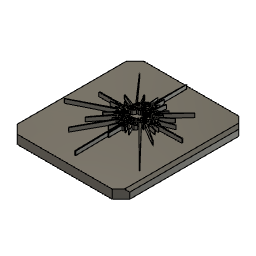
Plaque Nomai (Autodesk Fusion 360 design; units mm, degrees)
Autodesk Fusion 360 part; units mm, degrees
sketch "Sketch1" plane through (0, 0, 0) normal (0, 1, 0) x (1, 0, 0)
  line L0 (0, 0) -> (16, 0)
  line L1 (16, 0) -> (16, -18)
  line L2 (16, -18) -> (0, -18)
  line L3 (0, -18) -> (0, 0)
  constraint horizontal L0
  constraint vertical L1
  constraint horizontal L2
  constraint vertical L3
  constraint coincident L0.start L3.end
extrude "Extrude1" add sketch "Sketch1" along normal blind 3 contours L0 L1 L2 L3 picked at (5.333333, -12) makes body 1
sketch "Sketch2" plane through (0, 3, 0) normal (0, 1, 0) x (-1, 0, 0)
  line L0 (-3.5, 4) -> (-3.55, 4)
  line L1 (-3.55, 4) -> (-6.6, 7.39)
  line L2 (-6.6, 7.39) -> (-6.783242, 7.248473)
  line L3 (-6.783242, 7.248473) -> (-7.45, 7.248473)
  line L4 (-7.45, 7.248473) -> (-7.5, 7.45)
  line L5 (-7.5, 7.45) -> (-7.55, 7.45)
  line L6 (-7.55, 7.45) -> (-7.55, 7.15)
  line L7 (-7.55, 7.15) -> (-7.66975, 7.15)
  line L8 (-7.66975, 7.15) -> (-7.7, 7.6)
  line L9 (-7.7, 7.6) -> (-7.348129, 7.623653)
  line L10 (-7.348129, 7.623653) -> (-7.331455, 7.3756)
  line L11 (-7.331455, 7.3756) -> (-6.800321, 7.388831)
  line L12 (-6.800321, 7.388831) -> (-6.608305, 7.559685)
  line L13 (-6.608305, 7.559685) -> (-3.5, 4)
  line L14 (-6.2, 6.1) -> (-6.258087, 6.047739)
  line L15 (-6.258087, 6.047739) -> (-6.9, 7)
  line L16 (-6.9, 7) -> (-6.95, 7)
  line L17 (-6.95, 7) -> (-7.345894, 6.643813)
  line L18 (-7.345894, 6.643813) -> (-7.382435, 6.821906)
  line L19 (-7.382435, 6.821906) -> (-7.025574, 7.142976)
  line L20 (-7.025574, 7.142976) -> (-6.85, 7.142976)
  line L21 (-6.85, 7.142976) -> (-6.2, 6.1)
  line L22 (-7.191091, 7.142976) -> (-7.4, 7.142976)
  line L23 (-7.4, 7.142976) -> (-7.593291, 6.848491)
  line L24 (-7.593291, 6.848491) -> (-7.4, 5.527504)
  line L25 (-7.4, 5.527504) -> (-7.496646, 6.821906)
  line L26 (-7.496646, 6.821906) -> (-7.191091, 7.142976)
  line L27 (-7.609875, 7.047702) -> (-7.879433, 7.047702)
  line L28 (-7.879433, 7.047702) -> (-7.83, 2.2)
  line L29 (-7.83, 2.2) -> (-7.794916, 2.200358)
  line L30 (-7.794916, 2.200358) -> (-7.716057, 6.848491)
  line L31 (-7.716057, 6.848491) -> (-7.609875, 7.047702)
  line L32 (-8, 6.6) -> (-8.3, 6.6)
  line L33 (-8.3, 6.6) -> (-8.339414, 6.187997)
  line L34 (-8.339414, 6.187997) -> (-8.244092, 6.499241)
  line L35 (-8.244092, 6.499241) -> (-8.06588, 6.499241)
  line L36 (-8.06588, 6.499241) -> (-8.06588, 5.342936)
  line L37 (-8.06588, 5.342936) -> (-8, 5.342936)
  line L38 (-8, 5.342936) -> (-8, 6.6)
  line L39 (-8.438881, 7.087755) -> (-8.708271, 5.753238)
  line L40 (-8.708271, 5.753238) -> (-8.764863, 5.764661)
  line L41 (-8.764863, 5.764661) -> (-8.573576, 7.141633)
  line L42 (-8.573576, 7.141633) -> (-8.438881, 7.087755)
  line L43 (-8, 6.7) -> (-8.35, 6.7)
  line L44 (-8.35, 6.7) -> (-8.35, 7.2)
  line L45 (-8.35, 7.2) -> (-8.6, 7.2)
  line L46 (-8.6, 7.2) -> (-8.8, 6.95)
  line L47 (-8.8, 6.95) -> (-8.980246, 7.056907)
  line L48 (-8.980246, 7.056907) -> (-9.60392, 6.277315)
  line L49 (-9.60392, 6.277315) -> (-9.637964, 6.30455)
  line L50 (-9.637964, 6.30455) -> (-9.013716, 7.247048)
  line L51 (-9.013716, 7.247048) -> (-8.890123, 7.165188)
  line L52 (-8.890123, 7.165188) -> (-8.74056, 7.352142)
  line L53 (-8.74056, 7.352142) -> (-8.248844, 7.352142)
  line L54 (-8.248844, 7.352142) -> (-8.248844, 6.868399)
  line L55 (-8.248844, 6.868399) -> (-8, 6.868399)
  line L56 (-8, 6.868399) -> (-8, 6.7)
  line L57 (-8.001395, 6.96448) -> (-8.142811, 6.96448)
  line L58 (-8.142811, 6.96448) -> (-8.142811, 7.354078)
  line L59 (-8.142811, 7.354078) -> (-7.92088, 7.354078)
  line L60 (-7.92088, 7.354078) -> (-7.92088, 7.975797)
  line L61 (-7.92088, 7.975797) -> (-7.801013, 7.975797)
  line L62 (-7.801013, 7.975797) -> (-7.758384, 7.156414)
  line L63 (-7.758384, 7.156414) -> (-8, 7.156414)
  line L64 (-8, 7.156414) -> (-8.001395, 6.96448)
  line L65 (-8, 8.1) -> (-8.004849, 7.433169)
  line L66 (-8.004849, 7.433169) -> (-9.03, 7.41)
  line L67 (-9.03, 7.41) -> (-11.530001, 4.85)
  line L68 (-11.530001, 4.85) -> (-11.550001, 4.89)
  line L69 (-11.550001, 4.89) -> (-9.09, 7.54)
  line L70 (-9.09, 7.54) -> (-8.14, 7.56)
  line L71 (-8.14, 7.56) -> (-8.14, 8.15)
  line L72 (-8.14, 8.15) -> (-8, 8.1)
  line L73 (-8.25, 7.65) -> (-8.25, 8)
  line L74 (-8.25, 8) -> (-8.65, 7.65)
  line L75 (-8.65, 7.65) -> (-8.25, 7.65)
  line L76 (-8.25, 8.15) -> (-8.8, 7.65)
  line L77 (-8.8, 7.65) -> (-9.3, 8.15)
  line L78 (-9.3, 8.15) -> (-9.22, 8.25)
  line L79 (-9.22, 8.25) -> (-8.795, 7.825)
  line L80 (-8.795, 7.825) -> (-8.4375, 8.15)
  line L81 (-8.4375, 8.15) -> (-8.25, 8.15)
  line L82 (-8.4, 8.35) -> (-8.795, 7.955)
  line L83 (-8.795, 7.955) -> (-8.901457, 8.061457)
  line L84 (-8.901457, 8.061457) -> (-8.488611, 8.474303)
  line L85 (-8.488611, 8.474303) -> (-8.4, 8.35)
  line L86 (-8.546308, 8.555239) -> (-8.949047, 8.1525)
  line L87 (-8.949047, 8.1525) -> (-9.02, 8.21)
  line L88 (-9.02, 8.21) -> (-8.7, 8.55)
  line L89 (-8.7, 8.55) -> (-8.546308, 8.555239)
  line L90 (-9.075018, 7.787234) -> (-9.352052, 8.091971)
  line L91 (-9.352052, 8.091971) -> (-9.459599, 7.994201)
  line L92 (-9.459599, 7.994201) -> (-9.267314, 7.774446)
  line L93 (-9.267314, 7.774446) -> (-9.773316, 7.164174)
  line L94 (-9.773316, 7.164174) -> (-9.711912, 7.113262)
  line L95 (-9.711912, 7.113262) -> (-9.075018, 7.787234)
  line L96 (-8.945038, 7.644256) -> (-9.018767, 7.713929)
  line L97 (-9.018767, 7.713929) -> (-9.075018, 7.644256)
  line L98 (-9.075018, 7.644256) -> (-8.945038, 7.644256)
  line L99 (-8.8294, 8.584728) -> (-9.3, 8.584728)
  line L100 (-9.3, 8.584728) -> (-9.794941, 7.973993)
  line L101 (-9.794941, 7.973993) -> (-9.75, 7.75)
  line L102 (-9.75, 7.75) -> (-10.910001, 6.75)
  line L103 (-10.910001, 6.75) -> (-10.883433, 6.719182)
  line L104 (-10.883433, 6.719182) -> (-10.874451, 6.720984)
  line L105 (-9.54, 7.73) -> (-10.874451, 6.720984)
  line L106 (-9.54, 7.73) -> (-9.594657, 7.939603)
  line L107 (-9.594657, 7.939603) -> (-9.213535, 8.371845)
  line L108 (-9.213535, 8.371845) -> (-9.1, 8.28)
  line L109 (-9.1, 8.28) -> (-8.8294, 8.584728)
  line L110 (-9.757394, 8.193299) -> (-9.898058, 8.019727)
  line L111 (-9.898058, 8.019727) -> (-11.680001, 7.43)
  line L112 (-11.680001, 7.43) -> (-11.691706, 7.465371)
  line L113 (-11.691706, 7.465371) -> (-10.02, 8.13)
  line L114 (-10.02, 8.13) -> (-10.060088, 8.251131)
  line L115 (-10.060088, 8.251131) -> (-10.069408, 8.279292)
  line L116 (-10.069408, 8.279292) -> (-10.523963, 8.301132)
  line L117 (-10.523963, 8.301132) -> (-10.522401, 8.333643)
  line L118 (-10.522401, 8.333643) -> (-9.998681, 8.411924)
  line L119 (-9.998681, 8.411924) -> (-9.757394, 8.193299)
  line L120 (-9.696027, 8.279361) -> (-9.952526, 8.529848)
  line L121 (-9.952526, 8.529848) -> (-13.6, 8.5)
  line L122 (-13.6, 8.5) -> (-13.600686, 8.583817)
  line L123 (-13.600686, 8.583817) -> (-9.880537, 8.680784)
  line L124 (-9.880537, 8.680784) -> (-9.62, 8.38)
  line L125 (-9.62, 8.38) -> (-9.696027, 8.279361)
  line L126 (-9.479969, 8.54549) -> (-9.556698, 8.465692)
  line L127 (-9.556698, 8.465692) -> (-9.856172, 8.784172)
  line L128 (-9.856172, 8.784172) -> (-10.840001, 8.84)
  line L129 (-10.840001, 8.84) -> (-10.860001, 8.89)
  line L130 (-10.860001, 8.89) -> (-9.814413, 8.89)
  line L131 (-9.814413, 8.89) -> (-9.479969, 8.54549)
  line L132 (-9.518334, 8.758434) -> (-9.518334, 9.170027)
  line L133 (-9.518334, 9.170027) -> (-9.929882, 9.170027)
  line L134 (-9.929882, 9.170027) -> (-10.9, 9.4)
  line L135 (-10.9, 9.4) -> (-10.911903, 9.349787)
  line L136 (-10.911903, 9.349787) -> (-10, 9)
  line L137 (-10, 9) -> (-9.7, 9)
  line L138 (-9.7, 9) -> (-9.7, 8.939707)
  line L139 (-9.7, 8.939707) -> (-9.518334, 8.758434)
  line L140 (-8.537747, 8.691775) -> (-9.439601, 8.691775)
  line L141 (-9.439601, 8.691775) -> (-9.439601, 9.156301)
  line L142 (-9.439601, 9.156301) -> (-8.413887, 9.170027)
  line L143 (-8.537747, 8.691775) -> (-8.537747, 8.761446)
  line L144 (-8.537747, 8.761446) -> (-9.3, 8.8)
  line L145 (-9.3, 8.8) -> (-9.314788, 8.99633)
  line L146 (-9.314788, 8.99633) -> (-8.483616, 9.023874)
  line L147 (-8.483616, 9.023874) -> (-8.413887, 9.170027)
  line L148 (-8.523626, 8.940011) -> (-9.214555, 8.917115)
  line L149 (-9.214555, 8.917115) -> (-9.213155, 8.874853)
  line L150 (-9.213155, 8.874853) -> (-8.564151, 8.85507)
  line L151 (-8.564151, 8.85507) -> (-8.523626, 8.940011)
  line L152 (-8.459454, 9.588483) -> (-8.838801, 9.23942)
  line L153 (-8.838801, 9.23942) -> (-9.769123, 9.23942)
  line L154 (-9.769123, 9.23942) -> (-12.025575, 10.717433)
  line L155 (-12.025575, 10.717433) -> (-11.99598, 10.762616)
  line L156 (-11.99598, 10.762616) -> (-9.638536, 9.38846)
  line L157 (-9.638536, 9.38846) -> (-8.95, 9.38846)
  line L158 (-8.95, 9.38846) -> (-8.460762, 9.890243)
  line L159 (-8.460762, 9.890243) -> (-8.459454, 9.588483)
  line L160 (-8.95, 9.5) -> (-9.25, 9.5)
  line L161 (-9.25, 9.5) -> (-14.004695, 14.440687)
  line L162 (-14.004695, 14.440687) -> (-13.960001, 14.470001)
  line L163 (-13.960001, 14.470001) -> (-8.95, 9.5)
  line L164 (-9.415286, 9.5) -> (-9.554376, 9.5)
  line L165 (-9.554376, 9.5) -> (-9.590117, 9.537139)
  line L166 (-9.590117, 9.537139) -> (-9.554376, 9.595452)
  line L167 (-9.554376, 9.595452) -> (-9.415286, 9.5)
  line L168 (-8.5, 10) -> (-8.861207, 9.595452)
  line L169 (-8.861207, 9.595452) -> (-9.087752, 9.797726)
  line L170 (-9.087752, 9.797726) -> (-8.974479, 9.924589)
  line L171 (-8.974479, 9.924589) -> (-8.893129, 9.797726)
  line L172 (-8.893129, 9.797726) -> (-8.723811, 9.98736)
  line L173 (-8.723811, 9.98736) -> (-8.5, 10)
  line L174 (-8.515772, 9.833823) -> (-8.460762, 9.890243)
  line L175 (-8.350321, 9.702011) -> (-8.238397, 9.702496)
  line L176 (-8.238397, 9.702496) -> (-8.240191, 10.116471)
  line L177 (-8.240191, 10.116471) -> (-8.4, 10.2)
  line L178 (-8.4, 10.2) -> (-9.017739, 10.197322)
  line L179 (-9.017739, 10.197322) -> (-9.252195, 9.960979)
  line L180 (-9.252195, 9.960979) -> (-9.177243, 9.886625)
  line L181 (-9.177243, 9.886625) -> (-8.961542, 10.104062)
  line L182 (-8.961542, 10.104062) -> (-8.396178, 10.106512)
  line L183 (-8.396178, 10.106512) -> (-8.368597, 10.079151)
  line L184 (-8.368597, 10.079151) -> (-8.350321, 9.702011)
  line L185 (-8.320095, 10.48169) -> (-8.46955, 10.314302)
  line L186 (-8.46955, 10.314302) -> (-8.874608, 10.314302)
  line L187 (-8.874608, 10.314302) -> (-9.267118, 11.085337)
  line L188 (-9.267118, 11.085337) -> (-9.227774, 11.129402)
  line L189 (-9.227774, 11.129402) -> (-8.70887, 10.494309)
  line L190 (-8.70887, 10.494309) -> (-8.320095, 10.48169)
  line L191 (-8.218928, 10.594995) -> (-8.572943, 10.593461)
  line L192 (-8.572943, 10.593461) -> (-8.778364, 11.076791)
  line L193 (-8.778364, 11.076791) -> (-8.778648, 11.142484)
  line L194 (-8.778648, 11.142484) -> (-8.514482, 10.738211)
  line L195 (-8.514482, 10.738211) -> (-8.25, 10.7)
  line L196 (-8.25, 10.7) -> (-8.2, 10.75)
  line L197 (-8.2, 10.75) -> (-8.225, 12.675482)
  line L198 (-8.225, 12.675482) -> (-8.173235, 12.727247)
  line L199 (-8.173235, 12.727247) -> (-8.142708, 12.675482)
  line L200 (-8.142708, 12.675482) -> (-8.1, 10.7)
  line L201 (-8.1, 10.7) -> (-8.218928, 10.594995)
  line L202 (-8.329908, 10.828133) -> (-8.416009, 10.840573)
  line L203 (-8.416009, 10.840573) -> (-8.461558, 10.932274)
  line L204 (-8.461558, 10.932274) -> (-8.309915, 11.066163)
  line L205 (-8.309915, 11.066163) -> (-8.30891, 10.834353)
  line L206 (-8.30891, 10.834353) -> (-8.329908, 10.828133)
  line L207 (-8.05, 9.5) -> (-8.35, 9.5)
  line L208 (-8.35, 9.5) -> (-8.351472, 9.609975)
  line L209 (-8.351472, 9.609975) -> (-8.2, 9.609975)
  line L210 (-8.2, 9.609975) -> (-8.16102, 9.638167)
  line L211 (-8.16102, 9.638167) -> (-8.16102, 10.128527)
  line L212 (-8.16102, 10.128527) -> (-8.05, 10.25)
  line L213 (-8.05, 10.25) -> (-8.05, 9.5)
  line L214 (-7.7, 9.75) -> (-7.85, 9.75)
  line L215 (-7.85, 9.75) -> (-7.85, 9.35)
  line L216 (-7.85, 9.35) -> (-8.05, 9.35)
  line L217 (-8.05, 9.35) -> (-8.25, 9.25)
  line L218 (-8.25, 9.25) -> (-8.65, 9.25)
  line L219 (-8.65, 9.25) -> (-8.5, 9.4)
  line L220 (-8.5, 9.4) -> (-8, 9.4)
  line L221 (-8, 9.4) -> (-7.95, 9.4)
  line L222 (-7.95, 9.4) -> (-7.975, 9.93339)
  line L223 (-7.975, 9.93339) -> (-7.687787, 9.946851)
  line L224 (-7.687787, 9.946851) -> (-7.7, 9.75)
  line L225 (-8.23, 10.22) -> (-8.310655, 10.293715)
  line L226 (-8.310655, 10.293715) -> (-8.002551, 10.630825)
  line L227 (-8.002551, 10.630825) -> (-8.10551, 16.826528)
  line L228 (-8.10551, 16.826528) -> (-8.002551, 16.843181)
  line L229 (-8.002551, 16.843181) -> (-7.898695, 10.593466)
  line L230 (-7.898695, 10.593466) -> (-8.23, 10.22)
  line L231 (-7.713999, 9.524356) -> (-7.524068, 9.512573)
  line L232 (-7.524068, 9.512573) -> (-7.45, 9.55)
  line L233 (-7.45, 9.55) -> (-7.487034, 10.167916)
  line L234 (-7.487034, 10.167916) -> (-7.8, 10.167916)
  line L235 (-7.8, 10.167916) -> (-7.805924, 10.266755)
  line L236 (-7.805924, 10.266755) -> (-7.598199, 10.505373)
  line L237 (-7.598199, 10.505373) -> (-7.622996, 10.919112)
  line L238 (-7.622996, 10.919112) -> (-7.308455, 11.817933)
  line L239 (-7.308455, 11.817933) -> (-7.359161, 11.862073)
  line L240 (-7.359161, 11.862073) -> (-7.783134, 10.919112)
  line L241 (-7.783134, 10.919112) -> (-7.777477, 10.57874)
  line L242 (-7.777477, 10.57874) -> (-7.950623, 10.365557)
  line L243 (-7.950623, 10.365557) -> (-7.950623, 10.029722)
  line L244 (-7.950623, 10.029722) -> (-7.619829, 10.029722)
  line L245 (-7.619829, 10.029722) -> (-7.596455, 9.700116)
  line L246 (-7.596455, 9.700116) -> (-7.643517, 9.646055)
  line L247 (-7.643517, 9.646055) -> (-7.748004, 9.673086)
  line L248 (-7.748004, 9.673086) -> (-7.713999, 9.524356)
  line L249 (-7.266689, 10.801328) -> (-7.425065, 10.518635)
  line L250 (-7.425065, 10.518635) -> (-7.515354, 10.517134)
  line L251 (-7.515354, 10.517134) -> (-7.521353, 10.878116)
  line L252 (-7.521353, 10.878116) -> (-7.458429, 10.990431)
  line L253 (-7.458429, 10.990431) -> (-7.266689, 10.801328)
  line L254 (-7.324009, 10.180051) -> (-7.415948, 10.174541)
  line L255 (-7.415948, 10.174541) -> (-7.408061, 10.042959)
  line L256 (-7.408061, 10.042959) -> (-7.324009, 10.180051)
  line L257 (-7.256565, 10.290054) -> (-7.658368, 10.265973)
  line L258 (-7.658368, 10.265973) -> (-7.559894, 10.426586)
  line L259 (-7.559894, 10.426586) -> (-7.369978, 10.426586)
  line L260 (-7.369978, 10.426586) -> (-5.028617, 14.663257)
  line L261 (-5.028617, 14.663257) -> (-4.952926, 14.621427)
  line L262 (-4.952926, 14.621427) -> (-7.256565, 10.290054)
  line L263 (-6.70707, 9.928836) -> (-7.07594, 10.360941)
  line L264 (-7.07594, 10.360941) -> (-6.736052, 10.75616)
  line L265 (-6.736052, 10.75616) -> (-6.692551, 10.732119)
  line L266 (-6.692551, 10.732119) -> (-6.891505, 10.372115)
  line L267 (-6.891505, 10.372115) -> (-6.736052, 10.192315)
  line L268 (-6.736052, 10.192315) -> (-4.94439, 12.433038)
  line L269 (-4.94439, 12.433038) -> (-4.88337, 12.384247)
  line L270 (-4.88337, 12.384247) -> (-6.70707, 9.928836)
  line L271 (-6.793779, 9.85148) -> (-7.13334, 10.296614)
  line L272 (-7.13334, 10.296614) -> (-7.381747, 9.899896)
  line L273 (-7.381747, 9.899896) -> (-7.381747, 9.673954)
  line L274 (-7.381747, 9.673954) -> (-7.142356, 9.991348)
  line L275 (-7.142356, 9.991348) -> (-7.020449, 9.991348)
  line L276 (-7.020449, 9.991348) -> (-6.860763, 9.782014)
  line L277 (-6.860763, 9.782014) -> (-6.793779, 9.85148)
  line L278 (-7.001022, 9.77228) -> (-7.086487, 9.876932)
  line L279 (-7.086487, 9.876932) -> (-7.17544, 9.77228)
  line L280 (-7.17544, 9.77228) -> (-7.001022, 9.77228)
  line L281 (-6.955673, 9.665885) -> (-7.259161, 9.665885)
  line L282 (-7.259161, 9.665885) -> (-7.473218, 9.414054)
  line L283 (-7.473218, 9.414054) -> (-7.616719, 9.414054)
  line L284 (-7.616719, 9.414054) -> (-7.433925, 9.190225)
  line L285 (-7.433925, 9.190225) -> (-6.955673, 9.665885)
  line L286 (-6.912986, 8.743731) -> (-7.08835, 8.743731)
  line L287 (-7.08835, 8.743731) -> (-7.372875, 9.116716)
  line L288 (-7.372875, 9.116716) -> (-6.340812, 10.167916)
  line L289 (-6.340812, 10.167916) -> (-6.304563, 10.132326)
  line L290 (-6.304563, 10.132326) -> (-7.21139, 9.13331)
  line L291 (-7.21139, 9.13331) -> (-6.912986, 8.743731)
  line L292 (-6.991822, 9.023653) -> (-7.062188, 9.13331)
  line L293 (-7.062188, 9.13331) -> (-5.526816, 10.73213)
  line L294 (-5.526816, 10.73213) -> (-5.447724, 10.699562)
  line L295 (-5.447724, 10.699562) -> (-6.991822, 9.023653)
  line L296 (-6.332145, 9.149994) -> (-6.504112, 9.366822)
  line L297 (-6.504112, 9.366822) -> (-6.181909, 9.749665)
  line L298 (-6.181909, 9.749665) -> (-6.134688, 9.709924)
  line L299 (-6.134688, 9.709924) -> (-6.263304, 9.480284)
  line L300 (-6.263304, 9.480284) -> (-6.198996, 9.395012)
  line L301 (-6.198996, 9.395012) -> (-1.512701, 11.706599)
  line L302 (-1.512701, 11.706599) -> (-1.453789, 11.673604)
  line L303 (-1.453789, 11.673604) -> (-6.332145, 9.149994)
  line L304 (-6.356451, 8.991899) -> (-6.554758, 8.991899)
  line L305 (-6.554758, 8.991899) -> (-6.455604, 9.122101)
  line L306 (-6.455604, 9.122101) -> (-6.356451, 8.991899)
  line L307 (-6.518812, 9.2051) -> (-6.58988, 9.298423)
  line L308 (-6.58988, 9.298423) -> (-6.931342, 8.933809)
  line L309 (-6.931342, 8.933809) -> (-6.7859, 8.742824)
  line L310 (-6.7859, 8.742824) -> (-6.472631, 8.742824)
  line L311 (-6.472631, 8.742824) -> (-6.426449, 8.191167)
  line L312 (-6.426449, 8.191167) -> (-5.677298, 8.087203)
  line L313 (-5.677298, 8.087203) -> (-5.670084, 8.139185)
  line L314 (-5.670084, 8.139185) -> (-6.230753, 8.279842)
  line L315 (-6.230753, 8.279842) -> (-6.282735, 8.331824)
  line L316 (-6.282735, 8.331824) -> (-6.322485, 8.891394)
  line L317 (-6.322485, 8.891394) -> (-6.67107, 8.891394)
  line L318 (-6.67107, 8.891394) -> (-6.721523, 8.941847)
  line L319 (-6.721523, 8.941847) -> (-6.518812, 9.2051)
  line L320 (-6.198574, 8.853015) -> (-6.230074, 9.056679)
  line L321 (-6.230074, 9.056679) -> (-6.00852, 9.179764)
  line L322 (-6.00852, 9.179764) -> (-5.675418, 9.292362)
  line L323 (-5.675418, 9.292362) -> (-5.656496, 9.236383)
  line L324 (-5.656496, 9.236383) -> (-5.976238, 9.128302)
  line L325 (-5.976238, 9.128302) -> (-5.97898, 9.0296)
  line L326 (-5.97898, 9.0296) -> (-5.934998, 8.968057)
  line L327 (-5.934998, 8.968057) -> (-4.75305, 9.0296)
  line L328 (-4.75305, 9.0296) -> (-4.732247, 8.968057)
  line L329 (-4.732247, 8.968057) -> (-5.782043, 8.847434)
  line L330 (-5.782043, 8.847434) -> (-6.198574, 8.853015)
  line L331 (-6.19824, 8.577981) -> (-6.19824, 8.733432)
  line L332 (-6.19824, 8.733432) -> (-2.979053, 8.733432)
  line L333 (-2.979053, 8.733432) -> (-3.028301, 8.634935)
  line L334 (-3.028301, 8.634935) -> (-6.19824, 8.577981)
  line L335 (-6.085185, 8.486123) -> (-6.165266, 8.366002)
  line L336 (-6.165266, 8.366002) -> (-6.2044, 8.392092)
  line L337 (-6.2044, 8.392092) -> (-6.2044, 8.493189)
  line L338 (-6.2044, 8.493189) -> (-6.085185, 8.486123)
  line L339 (-6.538701, 8.139185) -> (-7.920849, 8.060711)
  line L340 (-7.920849, 8.060711) -> (-7.913393, 8.114433)
  line L341 (-7.913393, 8.114433) -> (-7.767998, 8.122688)
  line L342 (-7.767998, 8.122688) -> (-7.56644, 8.203089)
  line L343 (-7.56644, 8.203089) -> (-6.638651, 8.255766)
  line L344 (-6.638651, 8.255766) -> (-6.638651, 8.502975)
  line L345 (-6.638651, 8.502975) -> (-7.098117, 8.502975)
  line L346 (-7.098117, 8.502975) -> (-7.326312, 8.298875)
  line L347 (-7.326312, 8.298875) -> (-7.432077, 8.298875)
  line L348 (-7.432077, 8.298875) -> (-7.176933, 8.628046)
  line L349 (-7.176933, 8.628046) -> (-6.538911, 8.628046)
  line L350 (-6.538911, 8.628046) -> (-6.538701, 8.139185)
  line L351 (-6.741558, 8.354155) -> (-7.112023, 8.324075)
  line L352 (-7.112023, 8.324075) -> (-7.050278, 8.401651)
  line L353 (-7.050278, 8.401651) -> (-6.745308, 8.401651)
  line L354 (-6.745308, 8.401651) -> (-6.741558, 8.354155)
  line L355 (-7.435288, 7.734048) -> (-7.689555, 7.72082)
  line L356 (-7.689555, 7.72082) -> (-7.689555, 7.970611)
  line L357 (-7.689555, 7.970611) -> (-7.435288, 7.734048)
  line L358 (-7.53136, 7.980719) -> (-7.141879, 7.591238)
  line L359 (-7.141879, 7.591238) -> (-6.896712, 7.836405)
  line L360 (-6.896712, 7.836405) -> (-7.046394, 8.013512)
  line L361 (-7.046394, 8.013512) -> (-7.219282, 8.004517)
  line L362 (-7.219282, 8.004517) -> (-7.114342, 7.88035)
  line L363 (-7.114342, 7.88035) -> (-7.11062, 7.808808)
  line L364 (-7.11062, 7.808808) -> (-7.166812, 7.796483)
  line L365 (-7.166812, 7.796483) -> (-7.364654, 7.996174)
  line L366 (-7.364654, 7.996174) -> (-7.53136, 7.980719)
  line L367 (-6.811024, 7.922844) -> (-6.906945, 8.019661)
  line L368 (-6.906945, 8.019661) -> (-6.715435, 8.019661)
  line L369 (-6.715435, 8.019661) -> (-6.811024, 7.922844)
  line L370 (-6.863499, 7.49746) -> (-7.050562, 7.4928)
  line L371 (-7.050562, 7.4928) -> (-7.051445, 7.528226)
  line L372 (-7.051445, 7.528226) -> (-6.55325, 8.039342)
  line L373 (-6.55325, 8.039342) -> (-6.422113, 8.042609)
  line L374 (-6.422113, 8.042609) -> (-4.951084, 7.388831)
  line L375 (-4.951084, 7.388831) -> (-4.975732, 7.333372)
  line L376 (-4.975732, 7.333372) -> (-6.487681, 7.877484)
  line L377 (-6.487681, 7.877484) -> (-6.863499, 7.49746)
  constraint horizontal L0
  constraint parallel L0 L3
  constraint parallel L3 L5
  constraint perpendicular L5 L6
  constraint perpendicular L6 L7
  constraint perpendicular L8 L9
  constraint perpendicular L9 L10
  constraint perpendicular L1 L14
  constraint parallel L3 L16
  constraint parallel L14 L17
  constraint parallel L17 L19
  constraint parallel L16 L20
  constraint parallel L20 L22
  constraint parallel L7 L27
  constraint perpendicular L28 L29
  constraint parallel L27 L32
  constraint parallel L32 L35
  constraint perpendicular L35 L36
  constraint perpendicular L36 L37
  constraint perpendicular L32 L38
  constraint perpendicular L39 L40
  constraint horizontal L43
  constraint perpendicular L43 L44
  constraint perpendicular L44 L45
  constraint parallel L46 L48
  constraint perpendicular L46 L49
  constraint perpendicular L50 L51
  constraint parallel L46 L52
  constraint horizontal L53
  constraint perpendicular L53 L54
  constraint perpendicular L54 L55
  constraint perpendicular L43 L56
  constraint perpendicular L54 L57
  constraint perpendicular L57 L58
  constraint perpendicular L58 L59
  constraint perpendicular L59 L60
  constraint perpendicular L60 L61
  constraint perpendicular L60 L63
  constraint parallel L64 L65
  constraint vertical L71
  constraint perpendicular L7 L73
  constraint perpendicular L73 L75
  constraint parallel L77 L79
  constraint parallel L76 L80
  constraint horizontal L81
  constraint perpendicular L79 L82
  constraint perpendicular L82 L83
  constraint perpendicular L83 L84
  constraint parallel L84 L86
  constraint perpendicular L76 L90
  constraint perpendicular L90 L91
  constraint perpendicular L74 L92
  constraint perpendicular L93 L94
  constraint perpendicular L95 L96
  constraint horizontal L98
  constraint parallel L98 L99
  constraint perpendicular L87 L100
  constraint perpendicular L102 L103
  constraint perpendicular L101 L104
  constraint parallel L100 L110
  constraint perpendicular L111 L112
  constraint perpendicular L111 L114
  constraint perpendicular L111 L115
  constraint perpendicular L116 L117
  constraint perpendicular L67 L120
  constraint perpendicular L121 L122
  constraint horizontal L130
  constraint vertical L132
  constraint perpendicular L132 L133
  constraint perpendicular L134 L135
  constraint horizontal L137
  constraint perpendicular L137 L138
  constraint parallel L137 L140
  constraint perpendicular L140 L141
  constraint perpendicular L140 L143
  constraint parallel L146 L148
  constraint perpendicular L146 L149
  constraint horizontal L153
  constraint perpendicular L154 L155
  constraint parallel L153 L157
  constraint parallel L157 L160
  constraint parallel L160 L164
  constraint parallel L161 L165
  constraint perpendicular L168 L169
  constraint perpendicular L169 L170
  constraint parallel L168 L172
  constraint perpendicular L159 L175
  constraint perpendicular L175 L176
  constraint perpendicular L176 L178
  constraint perpendicular L163 L179
  constraint perpendicular L179 L180
  constraint perpendicular L163 L181
  constraint perpendicular L176 L182
  constraint perpendicular L179 L183
  constraint parallel L168 L185
  constraint horizontal L186
  constraint parallel L185 L188
  constraint parallel L178 L191
  constraint perpendicular L191 L193
  constraint parallel L196 L198
  constraint parallel L195 L202
  constraint parallel L201 L204
  constraint perpendicular L191 L205
  constraint perpendicular L71 L207
  constraint perpendicular L142 L208
  constraint perpendicular L71 L209
  constraint perpendicular L207 L211
  constraint perpendicular L207 L213
  constraint perpendicular L211 L214
  constraint perpendicular L214 L215
  constraint perpendicular L211 L216
  constraint perpendicular L211 L218
  constraint perpendicular L211 L220
  constraint perpendicular L211 L221
  constraint perpendicular L222 L223
  constraint perpendicular L212 L225
  constraint perpendicular L225 L226
  constraint parallel L227 L229
  constraint perpendicular L224 L231
  constraint perpendicular L213 L234
  constraint parallel L233 L235
  constraint parallel L235 L237
  constraint perpendicular L236 L239
  constraint parallel L229 L241
  constraint perpendicular L243 L244
  constraint parallel L236 L246
  constraint perpendicular L227 L250
  constraint perpendicular L250 L251
  constraint parallel L249 L252
  constraint perpendicular L233 L254
  constraint perpendicular L254 L255
  constraint perpendicular L233 L257
  constraint parallel L256 L258
  constraint horizontal L259
  constraint perpendicular L260 L261
  constraint perpendicular L260 L265
  constraint perpendicular L265 L266
  constraint perpendicular L268 L269
  constraint vertical L273
  constraint perpendicular L273 L275
  constraint parallel L271 L276
  constraint horizontal L280
  constraint parallel L280 L281
  constraint parallel L279 L282
  constraint parallel L281 L283
  constraint parallel L278 L284
  constraint parallel L234 L286
  constraint parallel L271 L287
  constraint perpendicular L288 L289
  constraint perpendicular L297 L298
  constraint perpendicular L299 L302
  constraint horizontal L304
  constraint parallel L306 L307
  constraint parallel L307 L309
  constraint horizontal L310
  constraint perpendicular L312 L313
  constraint parallel L310 L317
  constraint parallel L315 L318
  constraint perpendicular L322 L323
  constraint perpendicular L323 L324
  constraint perpendicular L322 L328
  constraint vertical L331
  constraint perpendicular L331 L332
  constraint perpendicular L335 L336
  constraint vertical L337
  constraint perpendicular L312 L340
  constraint parallel L339 L341
  constraint parallel L339 L343
  constraint vertical L344
  constraint perpendicular L344 L345
  constraint parallel L345 L347
  constraint parallel L347 L349
  constraint perpendicular L344 L353
  constraint perpendicular L62 L355
  constraint perpendicular L61 L356
  constraint perpendicular L358 L359
  constraint parallel L355 L361
  constraint parallel L360 L362
  constraint perpendicular L355 L363
  constraint parallel L365 L367
  constraint horizontal L368
  constraint parallel L11 L370
  constraint perpendicular L11 L371
  constraint parallel L370 L373
  constraint perpendicular L374 L375
extrude "Extrude2" add sketch "Sketch2" along normal blind 0.5 separate body contours L0 L1 L2 L3 L4 L5 L6 L7 L8 L9 L10 L11 L12 L13 | L14 L15 L16 L17 L18 L19 L20 L21 | L22 L23 L24 L25 L26 | L27 L28 L29 L30 L31 | L32 L33 L34 L35 L36 L37 L38 | L39 L40 L41 L42 | L43 L44 L45 L46 L47 L48 L49 L50 L51 L52 L53 L54 L55 L56 | L57 L58 L59 L60 L61 L62 L63 L64 | L65 L66 L67 L68 L69 L70 L71 L72 | L73 L74 L75 | L76 L77 L78 L79 L80 L81 | L82 L83 L84 L85 | L86 L87 L88 L89 | L90 L91 L92 L93 L94 L95 | L96 L97 L98 | L99 L100 L101 L102 L103 L104 L105 L106 L107 L108 L109 | L110 L111 L112 L113 L114 L115 L116 L117 L118 L119 | L120 L121 L122 L123 L124 L125 | L126 L127 L128 L129 L130 L131 | L132 L133 L134 L135 L136 L137 L138 L139 | L140 L141 L142 L143 L144 L145 L146 L147 | L148 L149 L150 L151 | L152 L153 L154 L155 L156 L157 L158 L159 L174 | L160 L161 L162 L163 | L164 L165 L166 L167 | L168 L169 L170 L171 L172 L173 | L175 L176 L177 L178 L179 L180 L181 L182 L183 L184 | L185 L186 L187 L188 L189 L190 | L191 L192 L193 L194 L195 L196 L197 L198 L199 L200 L201 | L202 L203 L204 L205 L206 | L207 L208 L209 L210 L211 L212 L213 | L214 L215 L216 L217 L218 L219 L220 L221 L222 L223 L224 | L225 L226 L227 L228 L229 L230 | L231 L232 L233 L234 L235 L236 L237 L238 L239 L240 L241 L242 L243 L244 L245 L246 L247 L248 | L249 L250 L251 L252 L253 | L254 L255 L256 | L257 L258 L259 L260 L261 L262 | L263 L264 L265 L266 L267 L268 L269 L270 | L271 L272 L273 L274 L275 L276 L277 | L278 L279 L280 | L281 L282 L283 L284 L285 | L286 L287 L288 L289 L290 L291 | L292 L293 L294 L295 | L296 L297 L298 L299 L300 L301 L302 L303 | L304 L305 L306 | L307 L308 L309 L310 L311 L312 L313 L314 L315 L316 L317 L318 L319 | L320 L321 L322 L323 L324 L325 L326 L327 L328 L329 L330 | L331 L332 L333 L334 | L335 L336 L337 L338 | L339 L340 L341 L342 L343 L344 L345 L346 L347 L348 L349 L350 | L351 L352 L353 L354 | L355 L356 L357 | L358 L359 L360 L361 L362 L363 L364 L365 L366 | L367 L368 L369 | L370 L371 L372 L373 L374 L375 L376 L377 picked at (-7.516043, 7.557884) picked at (-7.22611, 6.821906) picked at (-7.362579, 7.035952) picked at (-7.808497, 5.365398) picked at (-8.12196, 6.566414) picked at (-8.59244, 6.664683) picked at (-8.763374, 7.105063) picked at (-7.826759, 7.49543) picked at (-9.89, 6.613334) picked at (-8.383333, 7.766666) picked at (-8.965, 7.875) picked at (-8.596689, 8.295253) picked at (-8.731785, 8.419246) picked at (-9.231461, 7.884551) picked at (-9.012941, 7.66748) picked at (-9.114312, 8.513767) picked at (-10.532686, 7.859909) picked at (-11.144583, 8.59815) picked at (-10.170195, 8.838057) picked at (-10.276627, 9.190009) picked at (-9.056092, 9.107553) picked at (-8.767444, 8.904065) picked at (-10.46788, 9.796832) picked at (-10.72, 11.156667) picked at (-9.508012, 9.531817) picked at (-8.695006, 9.860937) picked at (-8.282395, 9.966039) picked at (-8.950199, 10.631316) picked at (-8.445808, 10.677224) picked at (-8.360128, 10.944263) picked at (-8.087007, 9.796055) picked at (-7.837596, 9.876747) picked at (-7.967933, 12.689157) picked at (-7.666224, 10.667742) picked at (-7.404369, 10.732693) picked at (-7.382672, 10.132517) picked at (-6.52649, 11.779356) picked at (-6.10883, 10.835133) picked at (-7.219148, 10.062619) picked at (-7.087649, 9.807164) picked at (-7.216253, 9.507332) picked at (-7.070909, 8.873591) picked at (-6.526942, 9.629698) picked at (-6.345084, 9.303943) picked at (-6.455604, 9.0353) picked at (-6.359284, 8.655347) picked at (-6.135876, 8.979765) picked at (-5.141594, 8.648783) picked at (-6.164662, 8.457135) picked at (-6.784832, 8.586355) picked at (-6.967953, 8.35996) picked at (-7.604799, 7.808493) picked at (-7.280017, 7.78948) picked at (-6.811134, 7.987388) picked at (-5.961842, 7.751155) makes body 2 at (8.753936, 3.166667, 8.932379) makes body 3 at (12.360636, 3.166667, 8.61614) makes body 4 at (9.097697, 3.166667, 9.160876) makes body 5 at (7.401533, 3.166667, 7.850892) makes body 6 at (5.720805, 3.166667, 13.177636) makes body 7 at (7.117301, 3.166667, 9.77228) makes body 8 at (3.079908, 3.166667, 10.8324) makes body 9 at (7.274508, 3.166667, 9.348778) makes body 10 at (9.429881, 3.166667, 6.618716) makes body 11 at (8.316666, 3.166667, 9.4) makes body 12 at (6.999417, 3.166667, 8.113027) makes body 13 at (8.433333, 3.166667, 7.983333) makes body 14 at (8.620402, 3.166667, 9.86515) makes body 15 at (8.05, 3.166667, 10) makes body 16 at (5.541015, 3.166667, 8.988572) makes body 17 at (8.30958, 3.166667, 10.988893) makes body 18 at (8.605913, 3.166667, 10.199107) makes body 19 at (10.730001, 3.166667, 5.773334) makes body 20 at (7.517354, 3.166667, 10.637462) makes body 21 at (7.967933, 3.166667, 14.759943) makes body 22 at (6.633333, 3.166667, 6.795317) makes body 23 at (8.701101, 3.166667, 6.223652) makes body 24 at (7.604799, 3.166667, 7.891757) makes body 25 at (8, 3.166667, 5.761957) makes body 26 at (10.511471, 3.166667, 8.89) makes body 27 at (9.031691, 3.166667, 7.644256) makes body 28 at (10.253254, 3.166667, 9.246685) makes body 29 at (9.005445, 3.166667, 10.571314) makes body 30 at (8.680554, 3.166667, 8.420993) makes body 31 at (5.572203, 3.166667, 6.373124) makes body 32 at (6.865046, 3.166667, 8.344129) makes body 33 at (7.862955, 3.166667, 5.431802) makes body 34 at (6.906966, 3.166667, 9.999858) makes body 35 at (7.028854, 3.166667, 9.467116) makes body 36 at (5.962423, 3.166667, 10.140926) makes body 37 at (5.125178, 3.166667, 8.733432) makes body 38 at (6.111879, 3.166667, 8.446083) makes body 39 at (12.29, 3.166667, 12.813334) makes body 40 at (6.422553, 3.166667, 8.991899) makes body 41 at (8.383333, 3.166667, 7.883333) makes body 42 at (8.763842, 3.166667, 8.199072) makes body 43 at (11.210165, 3.166667, 10.304564) makes body 44 at (6.176732, 3.166667, 8.156512) makes body 45 at (8.114236, 3.333333, 11.358494) makes body 46 at (9.508012, 3.166667, 9.563635) makes body 47 at (7.772594, 3.333333, 7.429542) makes body 48 at (7.500485, 3.166667, 11.547753) makes body 49 at (5.93177, 3.166667, 7.824683) makes body 50 at (6.843108, 3.166667, 8.019661) makes body 51 at (7.528861, 3.166667, 6.408162) makes body 52 at (7.380044, 3.166667, 10.088656) makes body 53 at (5.49127, 3.166667, 11.565777) makes body 54 at (10.492039, 3.166667, 7.823151) makes body 55 at (9.499614, 3.166667, 7.337919) makes body 56 at (9.984817, 3.166667, 7.393661)
scale "Scale1" factor 4 about (6.472631, 3.5, 8.742824) bodies 15 28 7 52 53 5 37 30 25 46 18 42 29 14 20 6 39 22 17 31 38 21 35 36 8 16 9 12 4 55 19 13 3 56 27 26 54 47 49 50 32 23 41 2 48 34 10 24 33 45 40 51 43 1 11 44
move_body "Move1" bodies 1 16 6 26 2 44 21 4 28 35 20 27 42 56 54 10 33 17 53 3 23 8 14 5 47 15 29 18 31 11 38 37 49 25 40 32 9 46 19 45 52 41 34 36 48 24 43 39 30 22 7 12 51 50 13 55 to x (1, 0, 0) y (0, 1, 0) z (0, 0, 1) at (25, 0, 30)
move_face "OffsetFaces1" offset -2 1 faces at (26.915441, 1.5, 27.771528) on bodies 1
move_body "Move2" bodies 18 2 13 53 19 16 41 23 7 20 33 14 46 9 15 43 39 21 6 45 28 37 31 8 48 56 3 44 12 30 42 54 4 52 29 38 36 35 27 32 50 55 34 10 26 17 5 49 47 22 11 25 24 51 40 to x (1, 0, 0) y (0, 1, 0) z (0, 0, 1) at (0, -2, 0)
scale "Scale2" factor 2 about (41.154625, -0.5, 42.962431) bodies 2 45 8 31 37 4 29 54 42 7 28 12 56 43 34 30 39 21 35 6 1 26 10 16 23 55 9 11 36 49 38 33 50 25 40 47 27 22 17 24 52 53 13 51 5 18 41 44 46 3 15 19 32 20 48 14
scale "Scale3" factor 1.1 about (41.221247, -0.5, 29.07228) bodies 6 31 43 48 11 22 53 9 40 35 17 44 20 15 49 36 52 25 34 8 51 33 19 46 45 21 14 39 7 29 38 18 37 28 16 4 23 56 5 50 2 54 3 30 10 27 47 26 13 32 41 12 55 24 42
move_face "OffsetFaces2" offset -10 1 faces at (12.676257, -0.5, 60.580625) on bodies 1
chamfer "Chamfer1" distance 10 angle 45 1 edges at (98.009591, -15.5, 108.580626) on bodies 1
chamfer "Chamfer2" distance 10 angle 45 1 edges at (98.009591, -15.5, -35.419376) on bodies 1
chamfer "Chamfer3" distance 10 angle 45 1 edges at (-29.990411, -15.5, -35.419376) on bodies 1
chamfer "Chamfer4" distance 10 angle 45 1 edges at (-29.990411, -15.5, 108.580626) on bodies 1
move_body "Move3" bodies 6 48 11 45 17 20 39 18 31 19 25 43 33 51 21 8 53 23 36 38 52 22 4 15 16 40 28 46 37 50 41 7 42 2 9 14 55 54 10 26 27 32 3 56 30 5 24 47 13 49 34 12 44 35 29 to x (1, 0, 0) y (0, 1, 0) z (0, 0, 1) at (0, -10, -10)
move_body "Move4" bodies 39 6 25 56 33 20 29 22 17 10 19 51 1 31 23 32 24 36 34 52 38 44 40 48 9 46 43 15 8 16 30 37 18 13 5 11 55 14 4 2 7 27 47 28 41 50 54 26 3 53 42 12 35 21 49 45 to x (1, 0, 0) y (0, 1, 0) z (0, 0, 1) at (40, 0, 40)
chamfer "Chamfer5" distance 3 angle 45 1 edges at (138.009591, -10.5, 76.580625) on bodies 1
